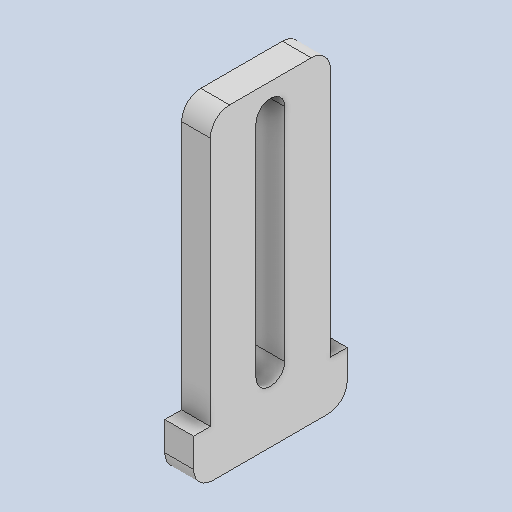
# Autodesk Inventor part: Ga motor 1
Saved by Autodesk Inventor 2023 (Build 270158000, 158)
## iProperties
Created: 2022-03-15
Part Number: Ga motor 1
Material: Generic
Document SubType Name: Modeling
Designer: phand
Density: 1 g/cm^3
Appearance: Default
Author: phand
Autodesk Inventor part; units mm, degrees
ref_plane "YZ Plane" through (0, 0, 0) normal (1, 0, 0) x (0, 1, 0)
ref_plane "XZ Plane" through (0, 0, 0) normal (0, 1, 0) x (-1, 0, 0)
ref_plane "XY Plane" through (0, 0, 0) normal (0, 0, 1) x (1, 0, 0)
sketch "Sketch1" plane through (0, 0, 0) normal (1, 0, 0) x (0, 1, 0)
  line L0 (-11.5722, 7.9995) -> (-14.5722, 7.9995)
  line L1 (-16.5722, 5.9995) -> (-16.5722, -5.9996)
  line L2 (-14.5722, -7.9996) -> (-11.5722, -7.9996)
  line L3 (16.4278, 8.0004) -> (-16.5722, -7.9996) construction
  line L4 (-11.5722, 7.9995) -> (-11.5722, 6.2495)
  line L5 (-11.5722, 6.2495) -> (14.4277, 6.2507)
  line L6 (-11.5722, -6.2496) -> (14.4277, -6.2508)
  line L7 (-11.5722, 7.9995) -> (-11.5722, 6.2495)
  line L8 (-11.5722, -6.2496) -> (-11.5722, -7.9996)
  arc A0 (-14.5722, 7.9995) -> (-16.5722, 5.9995) centre (-14.5722, 5.9995) ccw
  arc A1 (-16.5722, -5.9996) -> (-14.5722, -7.9996) centre (-14.5722, -5.9996) ccw
  line L9 (-16.5722, 7.9995) -> (-3.1229, 1.4787) construction
  line L10 (-2.3653, 1.1122) -> (16.4278, -7.9996) construction
  arc A2 (13.4, -1.5001) -> (13.4, 1.4999) centre (13.4, -0.0001) ccw
  arc A3 (-9.6, 1.4999) -> (-9.6, -1.4996) centre (-9.5722, 0.0001) ccw
  line L11 (13.4, 1.4999) -> (-9.6, 1.4999)
  line L12 (-9.6, -1.4996) -> (13.4, -1.5001)
  line L13 (16.4278, 4.2507) -> (16.4278, -4.2508)
  arc A4 (16.4278, 4.2507) -> (14.4277, 6.2507) centre (14.4278, 4.2507) ccw
  arc A5 (14.4277, -6.2508) -> (16.4278, -4.2508) centre (14.4278, -4.2508) ccw
  point P0 (16.4278, 6.2508)
  point P1 (16.4278, -6.2509)
  dimension "d1" = 16
  dimension "d3" = 1.75
  dimension "d5" = 2
  dimension "d14" = 1.75
  dimension "d18" = 3
  dimension "d19" = 3
  dimension "d21" = 2
  dimension "d24" = 28
  dimension "d25" = 2
  dimension "d26" = 5
  constraints: 28 end point, 12 point on circle, 10 tangent, 8 point on line, 6 centre point, 3 equal length, 3 perpendicular, 2 equal radius, 2 horizontal, 1 parallel, 1 vertical
  measures "d1" distance of L10.end L3.start
  measures "d3" distance of L0.start L4.end
  measures "d5" radius of A0
  measures "d14" distance of L6.start L2.end
  measures "d18" diameter of A2
  measures "d19" diameter of A3
  measures "d21" distance from line of L8 A3.centre
  measures "d24" distance of L4.end point (16.428, 6.251)
  measures "d25" radius of A4
  measures "d26" distance between parallel lines of L8 L1
extrude "Extrusion3" add sketch "Sketch1" along normal blind 3
body "Solid3"
